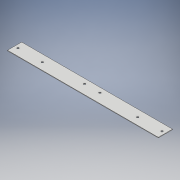
# Autodesk Inventor part: Линейка
Saved by Autodesk Inventor 2019.1 (Build 231200000, 200)
## iProperties
Created: 2018-02-13
Part Number: Линейка
Material: Типовые
Document SubType Name: Modeling
Designer: olege
Density: 1 g/cm^3
Appearance: По умолчанию
Mass: 8.90636 g
Surface Area: 156.474 cm^2
Volume: 8.90636 cm^3
Author: olege
Autodesk Inventor part; units mm, degrees
ref_plane "YZ Plane" through (0, 0, 0) normal (1, 0, 0) x (0, 1, 0)
ref_plane "XZ Plane" through (0, 0, 0) normal (0, 1, 0) x (-1, 0, 0)
ref_plane "XY Plane" through (0, 0, 0) normal (0, 0, 1) x (1, 0, 0)
sketch "Эскиз1" plane through (0, 0, 0) normal (0, 0, 1) x (1, 0, 0)
  line L0 (0, 0) -> (315, 0)
  line L1 (315, 0) -> (315, 29.5)
  line L2 (315, 29.5) -> (0, 29.5)
  line L3 (0, 29.5) -> (0, 0)
  dimension "d0" = 315
  dimension "d1" = 29.5
  constraints: 8 end point, 2 parallel, 1 horizontal, 1 perpendicular
  measures "d0" distance of L2.end L1.end
  measures "d1" distance of L1.end L0.end
extrude "Выдавливание1" add sketch "Эскиз1" along normal blind 1.2
sketch "Эскиз2" plane through (0, 0, 1.2) normal (0, 0, 1) x (1, 0, 0)
  circle A0 centre (58, 14.75) radius 2
  circle A1 centre (7, 14.75) radius 2
  point P0 (0, 0)
  constraints: 2 centre point, 4 other
extrude "Выдавливание2" cut sketch "Эскиз2" against normal blind 10
sketch "Эскиз4" plane through (0, 0, 1.2) normal (0, 0, 1) x (1, 0, 0)
  line L0 (315, 29.5) -> (0, 29.5) construction
  line L1 (157.5, 29.5) -> (157.5, 0) construction
  line L2 (0, 0) -> (315, 0) construction
  line L3 (157.5, 3.5) -> (173.5, 19.5) construction
  line L4 (173.5, 19.5) -> (157.5, 35.5) construction
  line L5 (157.5, 35.5) -> (141.5, 19.5) construction
  line L6 (141.5, 19.5) -> (157.5, 3.5) construction
  line L7 (157.5, 3.5) -> (157.5, 35.5) construction
  line L8 (173.5, 19.5) -> (141.5, 19.5) construction
  circle A0 centre (173.5, 19.5) radius 2
  circle A1 centre (141.5, 19.5) radius 2
  point P0 (157.5, 19.5)
  dimension "d11" = 4
  dimension "d12" = 4
  dimension "d15" = 32
  dimension "d16" = 10
  constraints: 14 end point, 3 midpoint, 2 centre point, 2 coincident, 2 parallel, 2 perpendicular, 2 point on line
  measures "d11" diameter of A0
  measures "d12" diameter of A1
  measures "d15" distance of L3.end L5.end
  measures "d16" distance between parallel lines of L0 L8
extrude "Выдавливание4" cut sketch "Эскиз4" against normal blind 10
sketch "Эскиз5" plane through (0, 0, 1.2) normal (0, 0, 1) x (1, 0, 0)
  circle A0 centre (308, 14.75) radius 2
  circle A1 centre (257, 14.75) radius 2
  point P0 (0, 0)
  constraints: 2 centre point, 4 other
extrude "Выдавливание5" cut sketch "Эскиз5" against normal blind 10
